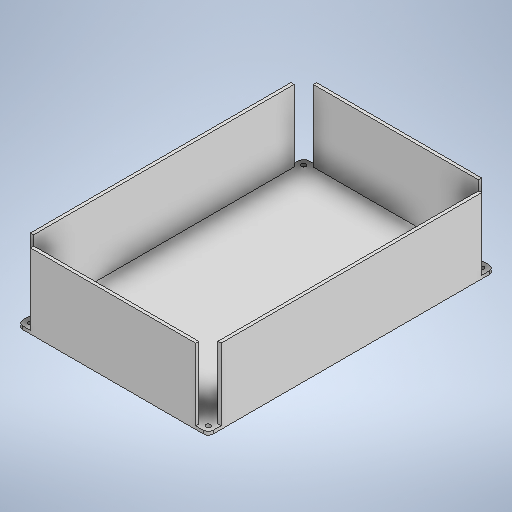
# Autodesk Inventor part: reduced_tortoise_base
Saved by Autodesk Inventor 2025.1 (Build 291241000, 241)
## iProperties
Created: 2025-04-09
Part Number: reduced_tortoise_base
Material: Generic
Document SubType Name: Modeling
Designer: Ian Ching
Density: 1 g/cm^3
Appearance: Default
Author: Ian Ching
Autodesk Inventor part; units mm, degrees
ref_plane "YZ Plane" through (0, 0, 0) normal (1, 0, 0) x (0, 1, 0)
ref_plane "XZ Plane" through (0, 0, 0) normal (0, 1, 0) x (-1, 0, 0)
ref_plane "XY Plane" through (0, 0, 0) normal (0, 0, 1) x (1, 0, 0)
sketch "Sketch1" plane through (0, 0, 0) normal (0, 1, 0) x (-1, 0, 0)
  line L0 (0, 0) -> (120, 0)
  line L1 (120, 0) -> (120, -180)
  line L2 (120, -180) -> (0, -180)
  line L3 (0, -180) -> (0, 0)
  dimension "d0" = 120
  dimension "d1" = 180
  constraints: 8 end point, 2 parallel, 1 horizontal, 1 perpendicular
  measures "d0" distance of L1.end L2.end
  measures "d1" distance of L0.end L1.end
extrude "Extrusion1" add sketch "Sketch1" along normal blind 2
sketch "Sketch2" plane through (0, 2, 0) normal (0, 1, 0) x (1, 0, 0)
  line L0 (-120, 0) -> (0, 0) projected
  line L1 (0, 0) -> (-8, 0)
  line L2 (-8, 0) -> (-8, 8)
  line L3 (-8, 8) -> (0, 8)
  line L4 (0, 8) -> (0, 0)
  line L5 (-120, 180) -> (-120, 0) projected
  line L6 (-120, 90) -> (0, 90)
  line L7 (0, 0) -> (0, 180) projected
  line L8 (-60, 0) -> (-60, 180)
  line L9 (0, 180) -> (-120, 180) projected
  line L10 (0, 180) -> (-8, 180)
  line L11 (-8, 180) -> (-8, 172)
  line L12 (-8, 172) -> (0, 172)
  line L13 (0, 172) -> (0, 180)
  line L14 (-120, 0) -> (-112, 0)
  line L15 (-112, 0) -> (-112, 8)
  line L16 (-112, 8) -> (-120, 8)
  line L17 (-120, 8) -> (-120, 0)
  line L18 (-120, 180) -> (-112, 180)
  line L19 (-112, 180) -> (-112, 172)
  line L20 (-112, 172) -> (-120, 172)
  line L21 (-120, 172) -> (-120, 180)
  line L22 (-120, 8) -> (-118, 8)
  line L23 (-118, 8) -> (-118, 172)
  line L24 (-118, 172) -> (-120, 172)
  line L25 (-120, 172) -> (-120, 8)
  line L26 (0, 172) -> (-2, 172)
  line L27 (-2, 172) -> (-2, 8)
  line L28 (-2, 8) -> (0, 8)
  line L29 (0, 8) -> (0, 172)
  line L30 (-8, 0) -> (-112, 0)
  line L31 (-112, 0) -> (-112, 2)
  line L32 (-112, 2) -> (-8, 2)
  line L33 (-8, 2) -> (-8, 0)
  line L34 (-8, 180) -> (-112, 180)
  line L35 (-112, 180) -> (-112, 178)
  line L36 (-112, 178) -> (-8, 178)
  line L37 (-8, 178) -> (-8, 180)
  point P0 (-8, 2)
  point P1 (-8, 178)
  dimension "d4" = 8
  dimension "d5" = 8
  dimension "d10" = 2
  dimension "d12" = 2
  dimension "d13" = 2
  dimension "d21" = 2
  constraints: 68 end point, 10 parallel, 9 symmetric about line, 5 horizontal, 5 perpendicular, 5 point on line, 4 midpoint
  measures "d4" distance of L2.end L3.end
  measures "d5" distance of L1.end L2.end
  measures "d10" distance of L24.end L23.end
  measures "d12" distance of L28.end L27.end
  measures "d13" distance of L30.end L31.end
  measures "d21" distance of L35.end L34.end
extrude "Extrusion2" add sketch "Sketch2" along normal blind 45 contours L15 L32 L8 L0 | L5 L6 L23 L16 | L8 L32 L2 L0 | L5 L20 L23 L6 | L3 L27 L6 L7 | L27 L12 L7 L6 | L36 L19 L9 L8 | L8 L9 L11 L36
sketch "Sketch4" plane through (0, 2, 0) normal (0, 1, 0) x (1, 0, 0)
  line L0 (0, 0) -> (-4, 0)
  line L1 (-4, 0) -> (-4, 4)
  line L2 (-4, 4) -> (0, 4)
  line L3 (0, 4) -> (0, 0)
  circle A0 centre (-4, 4) radius 1.5
  line L4 (-120, 180) -> (-120, 0) projected
  line L5 (-120, 90) -> (0, 90)
  line L6 (0, 8) -> (0, 180) projected
  line L7 (-120, 0) -> (0, 0) projected
  line L8 (-60, 0) -> (-60, 180)
  line L9 (0, 180) -> (-120, 180) projected
  circle A1 centre (-4, 176) radius 1.5
  circle A2 centre (-116, 4) radius 1.5
  circle A3 centre (-116, 176) radius 1.5
  point P0 (-120, 172)
  point P1 (-120, 8)
  point P2 (0, 172)
  dimension "d16" = 4
  dimension "d17" = 4
  dimension "d18" = 3
  constraints: 12 end point, 4 centre point, 3 midpoint, 3 symmetric about line, 2 parallel, 1 coincident, 1 horizontal, 1 perpendicular, 1 point on line, 3 other
  measures "d16" distance of L1.end L2.end
  measures "d17" distance of L0.end L1.end
  measures "d18" diameter of A0
extrude "Extrusion3" cut sketch "Sketch4" against normal blind 45 contours A0 L2 L1 | L1 L2 A0 | A1 | A2 | A3
fillet "Fillet1" radius 3 4 edges at (-120, 1, -180) (0, 1, -180) (-120, 1, 0) (0, 1, 0)
body "Solid1"
